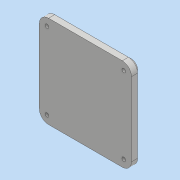
# Autodesk Inventor part: P8
Saved by Autodesk Inventor 2017 (Build 210142000, 142)
## iProperties
Part Number: P8
Material: 一般
Document SubType Name: Modeling
Designer: d8910
Density: 1 g/cm^3
Appearance: 預設
Author: d8910
Autodesk Inventor part; units mm, degrees
ref_plane "YZ Plane" through (0, 0, 0) normal (1, 0, 0) x (0, 1, 0)
ref_plane "XZ Plane" through (0, 0, 0) normal (0, 1, 0) x (-1, 0, 0)
ref_plane "XY Plane" through (0, 0, 0) normal (0, 0, 1) x (1, 0, 0)
sketch "草圖1" plane through (0, 0, 0) normal (0, 1, 0) x (-1, 0, 0)
  line L0 (120, 150) -> (-120, 150)
  line L1 (-150, 120) -> (-150, -120)
  line L2 (-120, -150) -> (120, -150)
  line L3 (150, -120) -> (150, 120)
  arc A0 (-120, 150) -> (-150, 120) centre (-120, 120) ccw
  arc A1 (150, 120) -> (120, 150) centre (120, 120) ccw
  arc A2 (120, -150) -> (150, -120) centre (120, -120) ccw
  arc A3 (-150, -120) -> (-120, -150) centre (-120, -120) ccw
  point P0 (0, 0)
  point P1 (150, 150)
  point P2 (150, -150)
  point P3 (150, 0)
  point P4 (0, -150)
  dimension "d0" = 300
  dimension "d1" = 30
  constraints: 8 end point, 8 point on circle, 8 tangent, 4 centre point, 4 point on line, 3 equal radius, 2 midpoint, 2 parallel, 2 perpendicular, 1 horizontal, 1 horizontal alignment, 1 vertical alignment
  measures "d0" distance of point (150, -150) point (150, 150)
  measures "d1" radius of A0
extrude "擠出1" add sketch "草圖1" along normal blind 30
chamfer "倒角1" distance 10 angle 45 8 edges at (150, 30, 0) (141.2132, 30, -141.2132) (0, 30, -150) (-141.2132, 30, -141.2132) (-150, 30, 0) (-141.2132, 30, 141.2132) (0, 30, 150) (141.2132, 30, 141.2132)
sketch "草圖2" plane through (0, 30, 0) normal (0, 1, 0) x (1, 0, 0)
  line L0 (140, 120) -> (140, -120) construction
  arc A0 (140, 120) -> (120, 140) centre (120, 120) ccw construction
  line L1 (-120, 140) -> (120, 140) construction
  arc A1 (-120, 140) -> (-140, 120) centre (-120, 120) ccw construction
  line L2 (-140, -120) -> (-140, 120) construction
  arc A2 (-140, -120) -> (-120, -140) centre (-120, -120) ccw construction
  line L3 (120, -140) -> (-120, -140) construction
  arc A3 (120, -140) -> (140, -120) centre (120, -120) ccw construction
  line L4 (-112.5, -112.5) -> (112.5, -112.5) construction
  line L5 (112.5, -112.5) -> (112.5, 112.5) construction
  line L6 (112.5, 112.5) -> (-112.5, 112.5) construction
  line L7 (-112.5, 112.5) -> (-112.5, -112.5) construction
  point P0 (0, 0)
  point P1 (-112.5, 0)
  point P2 (0, -112.5)
  dimension "d7" = 225
  constraints: 8 end point, 4 coincident, 2 midpoint, 2 parallel, 2 perpendicular, 1 horizontal, 1 horizontal alignment, 1 vertical alignment
  measures "d7" distance of L6.end L4.start
hole "孔1" at (-112.5, 30, 112.5) at (112.5, 30, 112.5) at (112.5, 30, -112.5) at (-112.5, 30, -112.5) direction (0, -1, 0) diameter 12 depth 10 tip angle 118
sketch "草圖3" plane through (0, 0, 0) normal (0, -1, 0) x (1, 0, 0)
  line L0 (125, 125) -> (-125, 125) construction
  line L1 (-125, 125) -> (-125, -125) construction
  line L2 (-125, -125) -> (125, -125) construction
  line L3 (125, -125) -> (125, 125) construction
  point P0 (0, 0)
  point P1 (125, 0)
  point P2 (0, -125)
  dimension "d15" = 250
  constraints: 8 end point, 4 coincident, 2 midpoint, 2 parallel, 2 perpendicular, 1 horizontal, 1 horizontal alignment, 1 vertical alignment
  measures "d15" distance of L2.end L0.start
hole "孔2" at (125, 0, 125) at (-125, 0, 125) at (-125, 0, -125) at (125, 0, -125) direction (0, 1, 0) diameter 12 depth 10 tip angle 118
